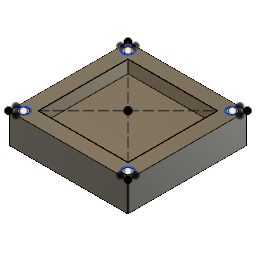
Bottom Part Enclosure (Autodesk Fusion 360 design; units mm, degrees)
Autodesk Fusion 360 part; units mm, degrees
sketch "Sketch1" plane through (0, 0, 0) normal (0, 1, 0) x (1, 0, 0)
  line L0 (40, -40) -> (-40, -40)
  line L1 (-40, -40) -> (-40, 40)
  line L2 (-40, 40) -> (40, 40)
  line L3 (40, 40) -> (40, -40)
  line L4 (40, -40) -> (-40, 40) construction
  line L5 (-40, -40) -> (40, 40) construction
  dimension "d1" = 80
  dimension "d2" = 80
extrude "Extrude1" add sketch "Sketch1" along normal blind 20
sketch "Sketch2" plane through (0, 20, 0) normal (0, 1, 0) x (-1, 0, 0)
  line L0 (-40, -40) -> (40, -40)
  line L1 (40, -40) -> (40, 40)
  line L2 (40, 40) -> (-40, 40)
  line L3 (-40, 40) -> (-40, -40)
  line L4 (40, -40) -> (35, -40)
  line L5 (-40, -40) -> (-35, -40)
  line L6 (40, -40) -> (40, -35)
  line L7 (-40, -40) -> (-40, -35)
  line L8 (40, 40) -> (40, 35)
  line L9 (40, 40) -> (35, 40)
  line L10 (-40, 40) -> (-40, 35)
  line L11 (-40, 40) -> (-35, 40)
  circle A0 centre (35, 35) radius 3.75
  circle A1 centre (-35, 35) radius 3.75
  circle A2 centre (35, -35) radius 3.75
  circle A3 centre (-35, -35) radius 3.75
  line L12 (-30, 30) -> (30, 30)
  line L13 (30, 30) -> (30, -30)
  line L14 (30, -30) -> (-30, -30)
  line L15 (-30, -30) -> (-30, 30)
  line L16 (-30, 30) -> (30, -30) construction
  line L17 (30, 30) -> (-30, -30) construction
  dimension "d5" = 5
  dimension "d6" = 5
  dimension "d7" = 5
  dimension "d8" = 5
  dimension "d9" = 5
  dimension "d10" = 5
  dimension "d11" = 5
  dimension "d12" = 5
  dimension "d13" = 7.5
  dimension "d14" = 7.5
  dimension "d15" = 7.5
  dimension "d16" = 7.5
  dimension "d25" = 60
  dimension "d26" = 60
  measures "d13" diameter of A0
  measures "d14" diameter of A1
  measures "d15" diameter of A2
  measures "d16" diameter of A3
extrude "Extrude6" cut sketch "Sketch2" against normal blind 8.5 contours L12 L13 L14 L15
extrude "Extrude2" cut sketch "Sketch2" against normal blind 5 contours A0
extrude "Extrude3" cut sketch "Sketch2" against normal blind 5 contours A2
extrude "Extrude4" cut sketch "Sketch2" against normal blind 5 contours A1
extrude "Extrude5" cut sketch "Sketch2" against normal blind 5 contours A3
thread "Thread1" "ISO Metric profile 7.0 M7x1 6H" major diameter 7.1472 minor diameter 6.0355 pitch 1 angle 60 resizes the face on face at (-38.7453, 16.6667, 34.8131)
thread "Thread2" "ISO Metric profile 7.0 M7x1 6H" major diameter 7.1472 minor diameter 6.0355 pitch 1 angle 60 resizes the face on face at (-38.7453, 16.6667, -35.1869)
thread "Thread3" "ISO Metric profile 7.0 M7x1 6H" major diameter 7.1472 minor diameter 6.0355 pitch 1 angle 60 resizes the face on face at (31.2547, 16.6667, 34.8131)
thread "Thread4" "ISO Metric profile 7.0 M7x1 6H" major diameter 7.1472 minor diameter 6.0355 pitch 1 angle 60 resizes the face on face at (31.2547, 16.6667, -35.1869)
fillet "Fillet1" radius 0.5 1 edges at (40, 10, 40)
fillet "Fillet2" radius 0.5 1 edges at (-40, 10, 40)
fillet "Fillet3" radius 0.5 1 edges at (40, 10, -40)
fillet "Fillet4" radius 0.5 1 edges at (-40, 10, -40)
